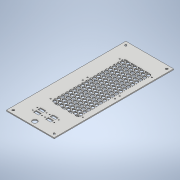
# Autodesk Inventor part: top_panel2
Saved by Autodesk Inventor 2022 (Build 260153000, 153)
## iProperties
Created: 2021-05-16
Part Number: top_panel2
Material: Generic
Document SubType Name: Modeling
Designer: gisen
Density: 1 g/cm^3
Appearance: Default
Author: gisen
Autodesk Inventor part; units mm, degrees
(part 1 of 2)
ref_plane "YZ Plane" through (0, 0, 0) normal (1, 0, 0) x (0, 1, 0)
ref_plane "XZ Plane" through (0, 0, 0) normal (0, 1, 0) x (-1, 0, 0)
ref_plane "XY Plane" through (0, 0, 0) normal (0, 0, 1) x (1, 0, 0)
sketch "Sketch1" plane through (0, 0, 0) normal (0, 0, 1) x (1, 0, 0)
  line L0 (-78, 195) -> (78, 195)
  line L1 (78, 195) -> (78, -195)
  line L2 (78, -195) -> (-78, -195)
  line L3 (-78, -195) -> (-78, 195)
  line L4 (-78, 195) -> (78, -195) construction
  line L5 (78, 195) -> (-78, -195) construction
  point P0 (0, 0)
  dimension "d1" = 156
  dimension "d2" = 390
  constraints: 12 end point, 2 midpoint, 2 parallel, 1 horizontal, 1 perpendicular
  measures "d1" distance of L0.start L0.end
  measures "d2" distance of L0.end L1.end
extrude "Extrusion1" add sketch "Sketch1" along normal blind 3
sketch "Sketch2" plane through (0, 0, 3) normal (0, 0, 1) x (1, 0, 0)
  line L0 (-78, -195) -> (78, -195) projected
  line L1 (-78, 195) -> (-78, -195) projected
  arc A0 (-64.4298, -185.2577) -> (-68.2577, -181.4298) centre (-66, -183) ccw
  arc A1 (-69.8472, -183.7153) -> (-66.7153, -186.8472) centre (-68, -185) ccw
  line L2 (-66.7153, -186.8472) -> (-64.4298, -185.2577)
  line L3 (-69.8472, -183.7153) -> (-68.2577, -181.4298)
  line L4 (0, 16.0888) -> (0, -25.3045)
  line L5 (-19.6832, 0) -> (22.709, 0)
  arc A2 (68.2577, -181.4298) -> (64.4298, -185.2577) centre (66, -183) ccw
  arc A3 (66.7153, -186.8472) -> (69.8472, -183.7153) centre (68, -185) ccw
  line L6 (66.7153, -186.8472) -> (64.4298, -185.2577)
  line L7 (69.8472, -183.7153) -> (68.2577, -181.4298)
  arc A4 (-68.2577, 181.4298) -> (-64.4298, 185.2577) centre (-66, 183) ccw
  arc A5 (-66.7153, 186.8472) -> (-69.8472, 183.7153) centre (-68, 185) ccw
  line L8 (-66.7153, 186.8472) -> (-64.4298, 185.2577)
  line L9 (-69.8472, 183.7153) -> (-68.2577, 181.4298)
  arc A6 (64.4298, 185.2577) -> (68.2577, 181.4298) centre (66, 183) ccw
  arc A7 (69.8472, 183.7153) -> (66.7153, 186.8472) centre (68, 185) ccw
  line L10 (66.7153, 186.8472) -> (64.4298, 185.2577)
  line L11 (69.8472, 183.7153) -> (68.2577, 181.4298)
  point P0 (0, 0)
  dimension "d11" = 12
  dimension "d12" = 10
  dimension "d13" = 12
  dimension "d14" = 10
  dimension "d15" = 5.5
  dimension "d16" = 4.5
  constraints: 24 symmetric about line, 20 end point, 16 point on circle, 8 centre point, 8 coincident, 4 tangent, 1 horizontal, 1 vertical, 6 other
  measures "d11" distance from line of L0 point (-66, -183)
  measures "d12" distance from line of L0 point (-68, -185)
  measures "d13" distance from line of L1 point (-66, -183)
  measures "d14" distance from line of L1 point (-68, -185)
  measures "d15" diameter of A0
  measures "d16" diameter of A1
extrude "Extrusion2" cut sketch "Sketch2" against normal up to surface (3 mm away)
sketch "Sketch4" plane through (0, 0, 3) normal (0, 0, 1) x (1, 0, 0)
  line L0 (-28.5, -132.4667) -> (-11.5, -132.4667)
  line L1 (-11.5, -132.4667) -> (-11.5, -141.4667)
  line L2 (-11.5, -141.4667) -> (-28.5, -141.4667)
  line L3 (-28.5, -141.4667) -> (-28.5, -132.4667)
  line L4 (-28.5, -132.4667) -> (-11.5, -141.4667) construction
  line L5 (-11.5, -132.4667) -> (-28.5, -141.4667) construction
  circle A0 centre (-35, -136.9667) radius 1.65
  circle A1 centre (-5, -136.9667) radius 1.65
  line L6 (0, -132.1595) -> (0, -155.449)
  line L7 (28.5, -132.4667) -> (11.5, -132.4667)
  line L8 (11.5, -132.4667) -> (11.5, -141.4667)
  line L9 (11.5, -141.4667) -> (28.5, -141.4667)
  line L10 (28.5, -141.4667) -> (28.5, -132.4667)
  line L11 (28.5, -132.4667) -> (11.5, -141.4667) construction
  line L12 (11.5, -132.4667) -> (28.5, -141.4667) construction
  circle A2 centre (35, -136.9667) radius 1.65
  circle A3 centre (5, -136.9667) radius 1.65
  line L13 (-30.7879, -144.4667) -> (-3.35, -144.4667)
  line L14 (-28.5, -156.4667) -> (-11.5, -156.4667)
  line L15 (-11.5, -156.4667) -> (-11.5, -147.4667)
  line L16 (-11.5, -147.4667) -> (-28.5, -147.4667)
  line L17 (-28.5, -147.4667) -> (-28.5, -156.4667)
  line L18 (-28.5, -156.4667) -> (-11.5, -147.4667) construction
  line L19 (-11.5, -156.4667) -> (-28.5, -147.4667) construction
  circle A4 centre (-35, -151.9667) radius 1.65
  circle A5 centre (-5, -151.9667) radius 1.65
  line L20 (28.5, -156.4667) -> (11.5, -156.4667)
  line L21 (11.5, -156.4667) -> (11.5, -147.4667)
  line L22 (11.5, -147.4667) -> (28.5, -147.4667)
  line L23 (28.5, -147.4667) -> (28.5, -156.4667)
  line L24 (28.5, -156.4667) -> (11.5, -147.4667) construction
  line L25 (11.5, -156.4667) -> (28.5, -147.4667) construction
  circle A6 centre (35, -151.9667) radius 1.65
  circle A7 centre (5, -151.9667) radius 1.65
  line L26 (-66.7153, 186.8472) -> (-64.4298, 185.2577) projected
  arc A8 (-68.2577, 181.4298) -> (-64.4298, 185.2577) centre (-66, 183) ccw projected
  line L27 (-68.2577, 181.4298) -> (-69.8472, 183.7153) projected
  arc A9 (-66.7153, 186.8472) -> (-69.8472, 183.7153) centre (-68, 185) ccw projected
  arc A10 (69.8472, 183.7153) -> (66.7153, 186.8472) centre (68, 185) ccw projected
  line L28 (69.8472, 183.7153) -> (68.2577, 181.4298) projected
  arc A11 (64.4298, 185.2577) -> (68.2577, 181.4298) centre (66, 183) ccw projected
  line L29 (64.4298, 185.2577) -> (66.7153, 186.8472) projected
  line L30 (66.7153, -186.8472) -> (64.4298, -185.2577) projected
  arc A12 (68.2577, -181.4298) -> (64.4298, -185.2577) centre (66, -183) ccw projected
  line L31 (68.2577, -181.4298) -> (69.8472, -183.7153) projected
  arc A13 (66.7153, -186.8472) -> (69.8472, -183.7153) centre (68, -185) ccw projected
  arc A14 (-69.8472, -183.7153) -> (-66.7153, -186.8472) centre (-68, -185) ccw projected
  line L32 (-69.8472, -183.7153) -> (-68.2577, -181.4298) projected
  arc A15 (-64.4298, -185.2577) -> (-68.2577, -181.4298) centre (-66, -183) ccw projected
  line L33 (-64.4298, -185.2577) -> (-66.7153, -186.8472) projected
  line L34 (78, 195) -> (-78, 195) projected
  line L35 (-78, 195) -> (-78, -195) projected
  line L36 (-78, -195) -> (78, -195) projected
  line L37 (78, -195) -> (78, 195) projected
  line L38 (78, -195) -> (-78, -195) projected
  point P0 (0, 0)
  point P1 (-20, -136.9667)
  point P2 (-5, -136.9667)
  point P3 (20, -136.9667)
  point P4 (-20, -151.9667)
  point P5 (20, -151.9667)
  point P6 (0, -195)
  dimension "d37" = 17
  dimension "d38" = 9
  dimension "d39" = 6.5
  dimension "d40" = 4.5
  dimension "d41" = 3.3
  dimension "d42" = 6.5
  dimension "d43" = 4.5
  dimension "d44" = 3.3
  dimension "d45" = 5
  dimension "d46" = 3
  dimension "d55" = 0
  constraints: 52 end point, 27 symmetric about line, 9 midpoint, 8 centre point, 8 coincident, 2 horizontal, 2 parallel, 1 perpendicular, 1 vertical, 6 other
  measures "d37" distance of L1.end L2.end
  measures "d38" distance of L0.end L1.end
  measures "d39" distance from line of L3 point (-35, -136.967)
  measures "d40" distance from line of point (-35, -136.967) L0
  measures "d41" diameter of A0
  measures "d42" distance from line of point (-5, -136.967) L1
  measures "d43" distance from line of L0 point (-5, -136.967)
  measures "d44" diameter of A1
  measures "d45" horizontal distance of A1.centre point (0, 0)
  measures "d46" distance between parallel lines of L13 L2
  measures "d55" distance from line of point (0, -195) L6
extrude "Extrusion4" cut sketch "Sketch4" against normal up to surface (3 mm away) contours L0 L1 L2 L3 | A0 | A1 | L10 L9 L8 L7 | A2 | A3 | L17 L16 L15 L14 | A4 | A5 | L20 L21 L22 L23 | A6 | A7
sketch "Sketch5" plane through (0, 0, 3) normal (0, 0, 1) x (1, 0, 0)
  line L0 (-78, -195) -> (78, -195) projected
  line L1 (-2.4755, -172.54) -> (2.4755, -172.54)
  line L2 (-2.4755, -187.46) -> (2.4755, -187.46)
  arc A0 (-2.4755, -172.54) -> (-2.4755, -187.46) centre (0, -180) ccw
  arc A1 (2.4755, -187.46) -> (2.4755, -172.54) centre (0, -180) ccw
  point P0 (0, 0)
  dimension "d49" = 15
  dimension "d51" = 7.46
  dimension "d52" = 7.46
  constraints: 4 end point, 4 point on circle, 2 centre point, 2 horizontal, 1 coincident
  measures "d49" distance from line of L0 point (0, -180)
  measures "d51" distance from line of A0.centre L1
  measures "d52" distance from line of point (0, -180) L2
extrude "Extrusion5" cut sketch "Sketch5" against normal up to surface (3 mm away)
sketch "Sketch7" plane through (0, 0, 3) normal (0, 0, 1) x (1, 0, 0)
  circle A0 centre (-38, -90.5) radius 2
  line L0 (-2.4755, -172.54) -> (2.4755, -172.54) projected
  arc A1 (2.4755, -187.46) -> (2.4755, -172.54) centre (0, -180) ccw projected
  line L1 (2.4755, -187.46) -> (-2.4755, -187.46) projected
  arc A2 (-2.4755, -172.54) -> (-2.4755, -187.46) centre (0, -180) ccw projected
  line L2 (-11.5, -156.4667) -> (-28.5, -156.4667) projected
  line L3 (-28.5, -156.4667) -> (-28.5, -147.4667) projected
  line L4 (-28.5, -147.4667) -> (-11.5, -147.4667) projected
  line L5 (-11.5, -147.4667) -> (-11.5, -156.4667) projected
  line L6 (11.5, -147.4667) -> (28.5, -147.4667) projected
  line L7 (28.5, -147.4667) -> (28.5, -156.4667) projected
  line L8 (28.5, -156.4667) -> (11.5, -156.4667) projected
  line L9 (11.5, -156.4667) -> (11.5, -147.4667) projected
  line L10 (11.5, -132.4667) -> (28.5, -132.4667) projected
  line L11 (28.5, -132.4667) -> (28.5, -141.4667) projected
  line L12 (28.5, -141.4667) -> (11.5, -141.4667) projected
  line L13 (11.5, -141.4667) -> (11.5, -132.4667) projected
  circle A3 centre (35, -151.9667) radius 1.65 projected
  circle A4 centre (-35, -151.9667) radius 1.65 projected
  circle A5 centre (5, -136.9667) radius 1.65 projected
  circle A6 centre (-5, -136.9667) radius 1.65 projected
  circle A7 centre (-35, -136.9667) radius 1.65 projected
  circle A8 centre (35, -136.9667) radius 1.65 projected
  circle A9 centre (-5, -151.9667) radius 1.65 projected
  circle A10 centre (5, -151.9667) radius 1.65 projected
  line L14 (-11.5, -132.4667) -> (-11.5, -141.4667) projected
  line L15 (-11.5, -141.4667) -> (-28.5, -141.4667) projected
  line L16 (-28.5, -141.4667) -> (-28.5, -132.4667) projected
  line L17 (-28.5, -132.4667) -> (-11.5, -132.4667) projected
  line L18 (-66.7153, 186.8472) -> (-64.4298, 185.2577) projected
  arc A11 (-68.2577, 181.4298) -> (-64.4298, 185.2577) centre (-66, 183) ccw projected
  line L19 (-68.2577, 181.4298) -> (-69.8472, 183.7153) projected
  arc A12 (-66.7153, 186.8472) -> (-69.8472, 183.7153) centre (-68, 185) ccw projected
  arc A13 (69.8472, 183.7153) -> (66.7153, 186.8472) centre (68, 185) ccw projected
  line L20 (69.8472, 183.7153) -> (68.2577, 181.4298) projected
  arc A14 (64.4298, 185.2577) -> (68.2577, 181.4298) centre (66, 183) ccw projected
  line L21 (64.4298, 185.2577) -> (66.7153, 186.8472) projected
  line L22 (66.7153, -186.8472) -> (64.4298, -185.2577) projected
  arc A15 (68.2577, -181.4298) -> (64.4298, -185.2577) centre (66, -183) ccw projected
  line L23 (68.2577, -181.4298) -> (69.8472, -183.7153) projected
  arc A16 (66.7153, -186.8472) -> (69.8472, -183.7153) centre (68, -185) ccw projected
  arc A17 (-69.8472, -183.7153) -> (-66.7153, -186.8472) centre (-68, -185) ccw projected
  line L24 (-69.8472, -183.7153) -> (-68.2577, -181.4298) projected
  arc A18 (-64.4298, -185.2577) -> (-68.2577, -181.4298) centre (-66, -183) ccw projected
  line L25 (-64.4298, -185.2577) -> (-66.7153, -186.8472) projected
  line L26 (78, 195) -> (-78, 195) projected
  line L27 (-78, 195) -> (-78, -195) projected
  line L28 (-78, -195) -> (78, -195) projected
  line L29 (78, -195) -> (78, 195) projected
  circle A19 centre (-38, 14.5) radius 2
  circle A20 centre (-38, 30) radius 2
  circle A21 centre (-38, 135) radius 2
  line L30 (14.5, 19.3358) -> (14.5, -21.6)
  circle A22 centre (67, -90.5) radius 2
  circle A23 centre (67, 14.5) radius 2
  circle A24 centre (67, 30) radius 2
  circle A25 centre (67, 135) radius 2
  point P0 (0, 0)
  dimension "d56" = 4
  dimension "d57" = 40
  dimension "d60" = 4
  dimension "d61" = 105
  dimension "d62" = 40
  dimension "d63" = 4
  dimension "d65" = 40
  dimension "d66" = 4
  dimension "d68" = 40
  dimension "d69" = 60
  dimension "d103" = 15.5
  dimension "d104" = 105
  dimension "d112" = 52.5
  constraints: 8 centre point, 4 symmetric about line, 2 end point, 1 vertical, 4 other
  measures "d56" diameter of A0
  measures "d57" distance from line of L27 A0.centre
  measures "d60" diameter of A19
  measures "d61" distance of A0.centre A19.centre
  measures "d62" distance from line of L27 A19.centre
  measures "d63" diameter of A20
  measures "d65" distance from line of L27 A20.centre
  measures "d66" diameter of A21
  measures "d68" distance from line of L27 A21.centre
  measures "d69" distance from line of L26 A21.centre
  measures "d103" distance of A19.centre A20.centre
  measures "d104" distance of A21.centre A20.centre
  measures "d112" distance from line of A19.centre L30
extrude "Extrusion7" cut sketch "Sketch7" against normal up to surface (3 mm away) contours A0 | A19 | A20 | A21 | A22 | A23 | A24 | A25
sketch "Sketch8" plane through (0, 0, 3) normal (0, 0, 1) x (1, 0, 0)
  circle A0 centre (-38, -90.5) radius 2 projected
  circle A1 centre (-38, 14.5) radius 2 projected
  circle A2 centre (67, 30) radius 2 projected
  circle A3 centre (67, 135) radius 2 projected
  circle A4 centre (67, -90.5) radius 2 projected
  circle A5 centre (67, 14.5) radius 2 projected
  circle A6 centre (-38, 30) radius 2 projected
  circle A7 centre (-38, 135) radius 2 projected
  line L0 (-2.4755, -172.54) -> (2.4755, -172.54) projected
  arc A8 (2.4755, -187.46) -> (2.4755, -172.54) centre (0, -180) ccw projected
  line L1 (2.4755, -187.46) -> (-2.4755, -187.46) projected
  arc A9 (-2.4755, -172.54) -> (-2.4755, -187.46) centre (0, -180) ccw projected
  line L2 (-11.5, -156.4667) -> (-28.5, -156.4667) projected
  line L3 (-28.5, -156.4667) -> (-28.5, -147.4667) projected
  line L4 (-28.5, -147.4667) -> (-11.5, -147.4667) projected
  line L5 (-11.5, -147.4667) -> (-11.5, -156.4667) projected
  line L6 (11.5, -147.4667) -> (28.5, -147.4667) projected
  line L7 (28.5, -147.4667) -> (28.5, -156.4667) projected
  line L8 (28.5, -156.4667) -> (11.5, -156.4667) projected
  line L9 (11.5, -156.4667) -> (11.5, -147.4667) projected
  line L10 (11.5, -132.4667) -> (28.5, -132.4667) projected
  line L11 (28.5, -132.4667) -> (28.5, -141.4667) projected
  line L12 (28.5, -141.4667) -> (11.5, -141.4667) projected
  line L13 (11.5, -141.4667) -> (11.5, -132.4667) projected
  circle A10 centre (35, -151.9667) radius 1.65 projected
  circle A11 centre (-35, -151.9667) radius 1.65 projected
  circle A12 centre (5, -136.9667) radius 1.65 projected
  circle A13 centre (-5, -136.9667) radius 1.65 projected
  circle A14 centre (-35, -136.9667) radius 1.65 projected
  circle A15 centre (35, -136.9667) radius 1.65 projected
  circle A16 centre (-5, -151.9667) radius 1.65 projected
  circle A17 centre (5, -151.9667) radius 1.65 projected
  line L14 (-11.5, -132.4667) -> (-11.5, -141.4667) projected
  line L15 (-11.5, -141.4667) -> (-28.5, -141.4667) projected
  line L16 (-28.5, -141.4667) -> (-28.5, -132.4667) projected
  line L17 (-28.5, -132.4667) -> (-11.5, -132.4667) projected
  line L18 (-66.7153, 186.8472) -> (-64.4298, 185.2577) projected
  arc A18 (-68.2577, 181.4298) -> (-64.4298, 185.2577) centre (-66, 183) ccw projected
  line L19 (-68.2577, 181.4298) -> (-69.8472, 183.7153) projected
  arc A19 (-66.7153, 186.8472) -> (-69.8472, 183.7153) centre (-68, 185) ccw projected
  arc A20 (69.8472, 183.7153) -> (66.7153, 186.8472) centre (68, 185) ccw projected
  line L20 (69.8472, 183.7153) -> (68.2577, 181.4298) projected
  arc A21 (64.4298, 185.2577) -> (68.2577, 181.4298) centre (66, 183) ccw projected
  line L21 (64.4298, 185.2577) -> (66.7153, 186.8472) projected
  line L22 (66.7153, -186.8472) -> (64.4298, -185.2577) projected
  arc A22 (68.2577, -181.4298) -> (64.4298, -185.2577) centre (66, -183) ccw projected
  line L23 (68.2577, -181.4298) -> (69.8472, -183.7153) projected
  arc A23 (66.7153, -186.8472) -> (69.8472, -183.7153) centre (68, -185) ccw projected
  arc A24 (-69.8472, -183.7153) -> (-66.7153, -186.8472) centre (-68, -185) ccw projected
  line L24 (-69.8472, -183.7153) -> (-68.2577, -181.4298) projected
  arc A25 (-64.4298, -185.2577) -> (-68.2577, -181.4298) centre (-66, -183) ccw projected
  line L25 (-64.4298, -185.2577) -> (-66.7153, -186.8472) projected
  line L26 (78, 195) -> (-78, 195) projected
  line L27 (-78, 195) -> (-78, -195) projected
  line L28 (-78, -195) -> (78, -195) projected
  line L29 (78, -195) -> (78, 195) projected
  circle A26 centre (-38, 135) radius 2 projected
  circle A27 centre (-38, 135) radius 6.33
  line L30 (-31.67, 135) -> (-31.67, 13.6115)
  arc A28 (-24.17, 142.5) -> (-31.67, 135) centre (-24.17, 135) ccw
  line L31 (-31.67, 13.6115) -> (-31.67, -90.5)
  arc A29 (-31.67, -90.5) -> (-24.17, -98) centre (-24.17, -90.5) ccw
  line L32 (-24.17, -98) -> (-10.2337, -98)
  line L33 (-24.17, 142.5) -> (-11.5, 142.5)
  line L34 (14.5, 11.7665) -> (14.5, -13.3152)
  line L35 (60.67, 135) -> (60.67, 13.6115)
  arc A30 (60.67, 135) -> (53.17, 142.5) centre (53.17, 135) ccw
  line L36 (60.67, 13.6115) -> (60.67, -90.5)
  arc A31 (53.17, -98) -> (60.67, -90.5) centre (53.17, -90.5) ccw
  line L37 (53.17, -98) -> (39.2337, -98)
  line L38 (53.17, 142.5) -> (40.5, 142.5)
  line L39 (40.5, 142.5) -> (-11.5, 142.5)
  line L40 (39.2337, -98) -> (12.6121, -98)
  circle A32 centre (-38, -90.5) radius 2 projected
  line L41 (-10.2337, -98) -> (21.6365, -98)
  line L42 (-21.286, -85.5048) -> (-27.054, -85.5048)
  line L43 (-27.054, -85.5048) -> (-29.9379, -90.5)
  line L44 (-29.9379, -90.5) -> (-27.054, -95.4952)
  line L45 (-27.054, -95.4952) -> (-21.286, -95.4952)
  line L46 (-21.286, -95.4952) -> (-18.4021, -90.5)
  line L47 (-18.4021, -90.5) -> (-21.286, -85.5048)
  line L48 (-7.1521, -84.0048) -> (-10.036, -89)
  line L49 (-10.036, -89) -> (-15.804, -89)
  line L50 (-15.804, -89) -> (-18.6879, -84.0048)
  line L51 (-7.1521, -96.9952) -> (-10.036, -92)
  line L52 (-10.036, -92) -> (-15.804, -92)
  line L53 (-15.804, -92) -> (-18.6879, -96.9952)
  line L54 (-1.67, -85.5048) -> (-4.554, -85.5048)
  line L55 (-4.554, -85.5048) -> (-7.4379, -90.5)
  line L56 (-7.4379, -90.5) -> (-4.554, -95.4952)
  line L57 (-4.554, -95.4952) -> (-1.67, -95.4952)
  line L58 (17.946, -85.5048) -> (20.83, -85.5048)
  line L59 (20.83, -95.4952) -> (17.946, -95.4952)
  line L60 (17.946, -95.4952) -> (15.0621, -90.5)
  line L61 (15.0621, -90.5) -> (17.946, -85.5048)
  line L62 (3.8121, -84.0048) -> (6.696, -89)
  line L63 (6.696, -89) -> (12.464, -89)
  line L64 (12.464, -89) -> (15.3479, -84.0048)
  line L65 (3.8121, -96.9952) -> (6.696, -92)
  line L66 (6.696, -92) -> (12.464, -92)
  line L67 (12.464, -92) -> (15.3479, -96.9952)
  line L68 (-1.67, -85.5048) -> (1.214, -85.5048)
  line L69 (1.214, -85.5048) -> (4.0979, -90.5)
  line L70 (4.0979, -90.5) -> (1.214, -95.4952)
  line L71 (1.214, -95.4952) -> (-1.67, -95.4952)
  line L72 (62.946, -95.4952) -> (60.0621, -90.5)
  line L73 (60.0621, -90.5) -> (62.946, -85.5048)
  line L74 (48.8121, -84.0048) -> (51.696, -89)
  line L75 (51.696, -89) -> (57.464, -89)
  line L76 (57.464, -89) -> (60.3479, -84.0048)
  line L77 (48.8121, -96.9952) -> (51.696, -92)
  line L78 (51.696, -92) -> (57.464, -92)
  line L79 (57.464, -92) -> (60.3479, -96.9952)
  line L80 (43.33, -85.5048) -> (46.214, -85.5048)
  line L81 (46.214, -85.5048) -> (49.0979, -90.5)
  line L82 (49.0979, -90.5) -> (46.214, -95.4952)
  line L83 (46.214, -95.4952) -> (43.33, -95.4952)
  line L84 (37.8479, -96.9952) -> (34.964, -92)
  line L85 (37.5621, -90.5) -> (40.446, -95.4952)
  line L86 (43.33, -85.5048) -> (40.446, -85.5048)
  line L87 (40.446, -85.5048) -> (37.5621, -90.5)
  line L88 (37.8479, -84.0048) -> (34.964, -89)
  line L89 (34.964, -92) -> (29.196, -92)
  line L90 (34.964, -89) -> (29.196, -89)
  line L91 (29.196, -92) -> (26.3121, -96.9952)
  line L92 (40.446, -95.4952) -> (43.33, -95.4952)
  line L93 (23.714, -95.4952) -> (26.5979, -90.5)
  line L94 (29.196, -89) -> (26.3121, -84.0048)
  line L95 (26.5979, -90.5) -> (23.714, -85.5048)
  line L96 (23.714, -85.5048) -> (20.83, -85.5048)
  line L97 (20.83, -95.4952) -> (23.714, -95.4952)
  line L98 (-21.286, -82.5048) -> (-27.054, -82.5048)
  line L99 (-27.054, -82.5048) -> (-29.9379, -77.5096)
  line L100 (-29.9379, -77.5096) -> (-27.054, -72.5144)
  line L101 (-27.054, -72.5144) -> (-21.286, -72.5144)
  line L102 (-21.286, -72.5144) -> (-18.4021, -77.5096)
  line L103 (-18.4021, -77.5096) -> (-21.286, -82.5048)
  line L104 (-7.1521, -84.0048) -> (-10.036, -79.0096)
  line L105 (-10.036, -79.0096) -> (-15.804, -79.0096)
  line L106 (-15.804, -79.0096) -> (-18.6879, -84.0048)
  line L107 (-7.1521, -71.0144) -> (-10.036, -76.0096)
  line L108 (-10.036, -76.0096) -> (-15.804, -76.0096)
  line L109 (-15.804, -76.0096) -> (-18.6879, -71.0144)
  line L110 (-1.67, -82.5048) -> (-4.554, -82.5048)
  line L111 (-4.554, -82.5048) -> (-7.4379, -77.5096)
  line L112 (-7.4379, -77.5096) -> (-4.554, -72.5144)
  line L113 (-4.554, -72.5144) -> (-1.67, -72.5144)
  line L114 (3.8121, -71.0144) -> (6.696, -76.0096)
  line L115 (4.0979, -77.5096) -> (1.214, -72.5144)
  line L116 (-1.67, -82.5048) -> (1.214, -82.5048)
  line L117 (1.214, -82.5048) -> (4.0979, -77.5096)
  line L118 (3.8121, -84.0048) -> (6.696, -79.0096)
  line L119 (6.696, -76.0096) -> (12.464, -76.0096)
  line L120 (6.696, -79.0096) -> (12.464, -79.0096)
  line L121 (12.464, -76.0096) -> (15.3479, -71.0144)
  line L122 (1.214, -72.5144) -> (-1.67, -72.5144)
  line L123 (17.946, -72.5144) -> (15.0621, -77.5096)
  line L124 (12.464, -79.0096) -> (15.3479, -84.0048)
  line L125 (15.0621, -77.5096) -> (17.946, -82.5048)
  line L126 (17.946, -82.5048) -> (20.83, -82.5048)
  line L127 (20.83, -72.5144) -> (17.946, -72.5144)
  line L128 (23.714, -82.5048) -> (20.83, -82.5048)
  line L129 (60.0621, -77.5096) -> (62.946, -82.5048)
  line L130 (57.464, -79.0096) -> (60.3479, -84.0048)
  line L131 (62.946, -72.5144) -> (60.0621, -77.5096)
  line L132 (57.464, -76.0096) -> (60.3479, -71.0144)
  line L133 (51.696, -76.0096) -> (57.464, -76.0096)
  line L134 (51.696, -79.0096) -> (57.464, -79.0096)
  line L135 (37.8479, -71.0144) -> (34.964, -76.0096)
  line L136 (34.964, -76.0096) -> (29.196, -76.0096)
  line L137 (34.964, -79.0096) -> (29.196, -79.0096)
  line L138 (37.8479, -84.0048) -> (34.964, -79.0096)
  line L139 (40.446, -82.5048) -> (37.5621, -77.5096)
  line L140 (37.5621, -77.5096) -> (40.446, -72.5144)
  line L141 (43.33, -82.5048) -> (40.446, -82.5048)
  line L142 (20.83, -72.5144) -> (23.714, -72.5144)
  line L143 (29.196, -76.0096) -> (26.3121, -71.0144)
  line L144 (23.714, -72.5144) -> (26.5979, -77.5096)
  line L145 (29.196, -79.0096) -> (26.3121, -84.0048)
  line L146 (26.5979, -77.5096) -> (23.714, -82.5048)
  line L147 (48.8121, -84.0048) -> (51.696, -79.0096)
  line L148 (48.8121, -71.0144) -> (51.696, -76.0096)
  line L149 (46.214, -82.5048) -> (49.0979, -77.5096)
  line L150 (49.0979, -77.5096) -> (46.214, -72.5144)
  line L151 (46.214, -72.5144) -> (43.33, -72.5144)
  line L152 (40.446, -72.5144) -> (43.33, -72.5144)
  line L153 (43.33, -82.5048) -> (46.214, -82.5048)
  line L154 (-32.969, -89.75) -> (-29.6521, -84.0048)
  line L155 (-29.6521, -84.0048) -> (-33.4021, -77.5096)
  line L156 (-33.4021, -77.5096) -> (-29.6521, -71.0144)
  line L157 (-21.286, -56.524) -> (-27.054, -56.524)
  line L158 (-27.054, -56.524) -> (-29.9379, -51.5289)
  line L159 (-29.9379, -51.5289) -> (-27.054, -46.5337)
  line L160 (-27.054, -46.5337) -> (-21.286, -46.5337)
  line L161 (-21.286, -46.5337) -> (-18.4021, -51.5289)
  line L162 (-18.4021, -51.5289) -> (-21.286, -56.524)
  line L163 (-7.1521, -58.024) -> (-10.036, -53.0289)
  line L164 (-10.036, -53.0289) -> (-15.804, -53.0289)
  line L165 (-15.804, -53.0289) -> (-18.6879, -58.024)
  line L166 (-7.1521, -45.0337) -> (-10.036, -50.0289)
  line L167 (-10.036, -50.0289) -> (-15.804, -50.0289)
  line L168 (-15.804, -50.0289) -> (-18.6879, -45.0337)
  line L169 (-1.67, -56.524) -> (-4.554, -56.524)
  line L170 (-4.554, -56.524) -> (-7.4379, -51.5289)
  line L171 (-7.4379, -51.5289) -> (-4.554, -46.5337)
  line L172 (-4.554, -46.5337) -> (-1.67, -46.5337)
  line L173 (3.8121, -45.0337) -> (6.696, -50.0289)
  line L174 (4.0979, -51.5289) -> (1.214, -46.5337)
  line L175 (-1.67, -56.524) -> (1.214, -56.524)
  line L176 (1.214, -56.524) -> (4.0979, -51.5289)
  line L177 (3.8121, -58.024) -> (6.696, -53.0289)
  line L178 (6.696, -50.0289) -> (12.464, -50.0289)
  line L179 (6.696, -53.0289) -> (12.464, -53.0289)
  line L180 (12.464, -50.0289) -> (15.3479, -45.0337)
  line L181 (1.214, -46.5337) -> (-1.67, -46.5337)
  line L182 (17.946, -46.5337) -> (15.0621, -51.5289)
  line L183 (12.464, -53.0289) -> (15.3479, -58.024)
  line L184 (15.0621, -51.5289) -> (17.946, -56.524)
  line L185 (17.946, -56.524) -> (20.83, -56.524)
  line L186 (20.83, -46.5337) -> (17.946, -46.5337)
  line L187 (23.714, -56.524) -> (20.83, -56.524)
  line L188 (60.0621, -51.5289) -> (62.946, -56.524)
  line L189 (57.464, -53.0289) -> (60.3479, -58.024)
  line L190 (62.946, -46.5337) -> (60.0621, -51.5289)
  line L191 (57.464, -50.0289) -> (60.3479, -45.0337)
  line L192 (51.696, -50.0289) -> (57.464, -50.0289)
  line L193 (51.696, -53.0289) -> (57.464, -53.0289)
  line L194 (37.8479, -45.0337) -> (34.964, -50.0289)
  line L195 (34.964, -50.0289) -> (29.196, -50.0289)
  line L196 (34.964, -53.0289) -> (29.196, -53.0289)
  line L197 (37.8479, -58.024) -> (34.964, -53.0289)
  line L198 (40.446, -56.524) -> (37.5621, -51.5289)
  line L199 (37.5621, -51.5289) -> (40.446, -46.5337)
  line L200 (43.33, -56.524) -> (40.446, -56.524)
  line L201 (20.83, -46.5337) -> (23.714, -46.5337)
  line L202 (29.196, -50.0289) -> (26.3121, -45.0337)
  line L203 (23.714, -46.5337) -> (26.5979, -51.5289)
  line L204 (29.196, -53.0289) -> (26.3121, -58.024)
  line L205 (26.5979, -51.5289) -> (23.714, -56.524)
  line L206 (48.8121, -58.024) -> (51.696, -53.0289)
  line L207 (48.8121, -45.0337) -> (51.696, -50.0289)
  line L208 (46.214, -56.524) -> (49.0979, -51.5289)
  line L209 (49.0979, -51.5289) -> (46.214, -46.5337)
  line L210 (46.214, -46.5337) -> (43.33, -46.5337)
  line L211 (40.446, -46.5337) -> (43.33, -46.5337)
  line L212 (43.33, -56.524) -> (46.214, -56.524)
  line L213 (-18.4021, -64.5192) -> (-21.286, -59.524)
  line L214 (-21.286, -69.5144) -> (-18.4021, -64.5192)
  line L215 (-27.054, -69.5144) -> (-21.286, -69.5144)
  line L216 (-21.286, -59.524) -> (-27.054, -59.524)
  line L217 (-15.804, -66.0192) -> (-18.6879, -71.0144)
  line L218 (-10.036, -66.0192) -> (-15.804, -66.0192)
  line L219 (-10.036, -63.0192) -> (-15.804, -63.0192)
  line L220 (-7.1521, -71.0144) -> (-10.036, -66.0192)
  line L221 (-7.4379, -64.5192) -> (-4.554, -69.5144)
  line L222 (-7.1521, -58.024) -> (-10.036, -63.0192)
  line L223 (-4.554, -59.524) -> (-7.4379, -64.5192)
  line L224 (-15.804, -63.0192) -> (-18.6879, -58.024)
  line L225 (-1.67, -59.524) -> (-4.554, -59.524)
  line L226 (-4.554, -69.5144) -> (-1.67, -69.5144)
  line L227 (1.214, -69.5144) -> (-1.67, -69.5144)
  line L228 (-1.67, -59.524) -> (1.214, -59.524)
  line L229 (4.0979, -64.5192) -> (1.214, -69.5144)
  line L230 (3.8121, -71.0144) -> (6.696, -66.0192)
  line L231 (1.214, -59.524) -> (4.0979, -64.5192)
  line L232 (3.8121, -58.024) -> (6.696, -63.0192)
  line L233 (17.946, -59.524) -> (20.83, -59.524)
  line L234 (12.464, -63.0192) -> (15.3479, -58.024)
  line L235 (6.696, -63.0192) -> (12.464, -63.0192)
  line L236 (15.0621, -64.5192) -> (17.946, -59.524)
  line L237 (6.696, -66.0192) -> (12.464, -66.0192)
  line L238 (17.946, -69.5144) -> (15.0621, -64.5192)
  line L239 (12.464, -66.0192) -> (15.3479, -71.0144)
  line L240 (20.83, -69.5144) -> (17.946, -69.5144)
  line L241 (51.696, -63.0192) -> (57.464, -63.0192)
  line L242 (51.696, -66.0192) -> (57.464, -66.0192)
  line L243 (20.83, -69.5144) -> (23.714, -69.5144)
  line L244 (23.714, -59.524) -> (20.83, -59.524)
  line L245 (23.714, -69.5144) -> (26.5979, -64.5192)
  line L246 (26.5979, -64.5192) -> (23.714, -59.524)
  line L247 (29.196, -63.0192) -> (26.3121, -58.024)
  line L248 (29.196, -66.0192) -> (26.3121, -71.0144)
  line L249 (34.964, -63.0192) -> (29.196, -63.0192)
  line L250 (34.964, -66.0192) -> (29.196, -66.0192)
  line L251 (37.8479, -58.024) -> (34.964, -63.0192)
  line L252 (37.8479, -71.0144) -> (34.964, -66.0192)
  line L253 (48.8121, -71.0144) -> (51.696, -66.0192)
  line L254 (48.8121, -58.024) -> (51.696, -63.0192)
  line L255 (46.214, -59.524) -> (49.0979, -64.5192)
  line L256 (49.0979, -64.5192) -> (46.214, -69.5144)
  line L257 (43.33, -59.524) -> (46.214, -59.524)
  line L258 (46.214, -69.5144) -> (43.33, -69.5144)
  line L259 (43.33, -59.524) -> (40.446, -59.524)
  line L260 (40.446, -59.524) -> (37.5621, -64.5192)
  line L261 (40.446, -69.5144) -> (43.33, -69.5144)
  line L262 (37.5621, -64.5192) -> (40.446, -69.5144)
  line L263 (57.464, -66.0192) -> (60.3479, -71.0144)
  line L264 (57.464, -63.0192) -> (60.3479, -58.024)
  line L265 (60.0621, -64.5192) -> (62.946, -59.524)
  line L266 (62.946, -69.5144) -> (60.0621, -64.5192)
  line L267 (-27.054, -59.524) -> (-29.9379, -64.5192)
  line L268 (-29.9379, -64.5192) -> (-27.054, -69.5144)
  line L269 (-32.969, -52.2789) -> (-29.6521, -58.024)
  line L270 (-29.6521, -58.024) -> (-33.4021, -64.5192)
  line L271 (-33.4021, -64.5192) -> (-29.6521, -71.0144)
  line L272 (-21.286, -4.5625) -> (-27.054, -4.5625)
  line L273 (-27.054, -4.5625) -> (-29.9379, 0.4327)
  line L274 (-29.9379, 0.4327) -> (-27.054, 5.4279)
  line L275 (-27.054, 5.4279) -> (-21.286, 5.4279)
  line L276 (-21.286, 5.4279) -> (-18.4021, 0.4327)
  line L277 (-18.4021, 0.4327) -> (-21.286, -4.5625)
  line L278 (-7.1521, -6.0625) -> (-10.036, -1.0673)
  line L279 (-10.036, -1.0673) -> (-15.804, -1.0673)
  line L280 (-15.804, -1.0673) -> (-18.6879, -6.0625)
  line L281 (-7.1521, 6.9279) -> (-10.036, 1.9327)
  line L282 (-10.036, 1.9327) -> (-15.804, 1.9327)
  line L283 (-15.804, 1.9327) -> (-18.6879, 6.9279)
  line L284 (-1.67, -4.5625) -> (-4.554, -4.5625)
  line L285 (-4.554, -4.5625) -> (-7.4379, 0.4327)
  line L286 (-7.4379, 0.4327) -> (-4.554, 5.4279)
  line L287 (-4.554, 5.4279) -> (-1.67, 5.4279)
  line L288 (3.8121, 6.9279) -> (6.696, 1.9327)
  line L289 (4.0979, 0.4327) -> (1.214, 5.4279)
  line L290 (-1.67, -4.5625) -> (1.214, -4.5625)
  line L291 (1.214, -4.5625) -> (4.0979, 0.4327)
  line L292 (3.8121, -6.0625) -> (6.696, -1.0673)
  line L293 (6.696, 1.9327) -> (12.464, 1.9327)
  line L294 (6.696, -1.0673) -> (12.464, -1.0673)
  line L295 (12.464, 1.9327) -> (15.3479, 6.9279)
  line L296 (1.214, 5.4279) -> (-1.67, 5.4279)
  line L297 (17.946, 5.4279) -> (15.0621, 0.4327)
  line L298 (12.464, -1.0673) -> (15.3479, -6.0625)
  line L299 (15.0621, 0.4327) -> (17.946, -4.5625)
  line L300 (17.946, -4.5625) -> (20.83, -4.5625)
  line L301 (20.83, 5.4279) -> (17.946, 5.4279)
  line L302 (23.714, -4.5625) -> (20.83, -4.5625)
  line L303 (60.0621, 0.4327) -> (62.946, -4.5625)
  line L304 (57.464, -1.0673) -> (60.3479, -6.0625)
  line L305 (62.946, 5.4279) -> (60.0621, 0.4327)
  line L306 (57.464, 1.9327) -> (60.3479, 6.9279)
  line L307 (51.696, 1.9327) -> (57.464, 1.9327)
  line L308 (51.696, -1.0673) -> (57.464, -1.0673)
  line L309 (37.8479, 6.9279) -> (34.964, 1.9327)
  line L310 (34.964, 1.9327) -> (29.196, 1.9327)
  line L311 (34.964, -1.0673) -> (29.196, -1.0673)
  line L312 (37.8479, -6.0625) -> (34.964, -1.0673)
  line L313 (40.446, -4.5625) -> (37.5621, 0.4327)
  line L314 (37.5621, 0.4327) -> (40.446, 5.4279)
  line L315 (43.33, -4.5625) -> (40.446, -4.5625)
  line L316 (20.83, 5.4279) -> (23.714, 5.4279)
  line L317 (29.196, 1.9327) -> (26.3121, 6.9279)
  line L318 (23.714, 5.4279) -> (26.5979, 0.4327)
  line L319 (29.196, -1.0673) -> (26.3121, -6.0625)
  line L320 (26.5979, 0.4327) -> (23.714, -4.5625)
  line L321 (48.8121, -6.0625) -> (51.696, -1.0673)
  line L322 (48.8121, 6.9279) -> (51.696, 1.9327)
  line L323 (46.214, -4.5625) -> (49.0979, 0.4327)
  line L324 (49.0979, 0.4327) -> (46.214, 5.4279)
  line L325 (46.214, 5.4279) -> (43.33, 5.4279)
  line L326 (40.446, 5.4279) -> (43.33, 5.4279)
  line L327 (43.33, -4.5625) -> (46.214, -4.5625)
  line L328 (-18.4021, -12.5577) -> (-21.286, -7.5625)
  line L329 (-21.286, -17.5529) -> (-18.4021, -12.5577)
  line L330 (-27.054, -17.5529) -> (-21.286, -17.5529)
  line L331 (-21.286, -7.5625) -> (-27.054, -7.5625)
  line L332 (-15.804, -14.0577) -> (-18.6879, -19.0529)
  line L333 (-10.036, -14.0577) -> (-15.804, -14.0577)
  line L334 (-10.036, -11.0577) -> (-15.804, -11.0577)
  line L335 (-7.1521, -19.0529) -> (-10.036, -14.0577)
  line L336 (-7.4379, -12.5577) -> (-4.554, -17.5529)
  line L337 (-7.1521, -6.0625) -> (-10.036, -11.0577)
  line L338 (-4.554, -7.5625) -> (-7.4379, -12.5577)
  line L339 (-15.804, -11.0577) -> (-18.6879, -6.0625)
  line L340 (-1.67, -7.5625) -> (-4.554, -7.5625)
  line L341 (-4.554, -17.5529) -> (-1.67, -17.5529)
  line L342 (1.214, -17.5529) -> (-1.67, -17.5529)
  line L343 (-1.67, -7.5625) -> (1.214, -7.5625)
  line L344 (4.0979, -12.5577) -> (1.214, -17.5529)
  line L345 (3.8121, -19.0529) -> (6.696, -14.0577)
  line L346 (1.214, -7.5625) -> (4.0979, -12.5577)
  line L347 (3.8121, -6.0625) -> (6.696, -11.0577)
  line L348 (17.946, -7.5625) -> (20.83, -7.5625)
  line L349 (12.464, -11.0577) -> (15.3479, -6.0625)
  line L350 (6.696, -11.0577) -> (12.464, -11.0577)
  line L351 (15.0621, -12.5577) -> (17.946, -7.5625)
  line L352 (6.696, -14.0577) -> (12.464, -14.0577)
  line L353 (17.946, -17.5529) -> (15.0621, -12.5577)
  line L354 (12.464, -14.0577) -> (15.3479, -19.0529)
  line L355 (20.83, -17.5529) -> (17.946, -17.5529)
  line L356 (51.696, -11.0577) -> (57.464, -11.0577)
  line L357 (51.696, -14.0577) -> (57.464, -14.0577)
  line L358 (20.83, -17.5529) -> (23.714, -17.5529)
  line L359 (23.714, -7.5625) -> (20.83, -7.5625)
  line L360 (23.714, -17.5529) -> (26.5979, -12.5577)
  line L361 (26.5979, -12.5577) -> (23.714, -7.5625)
  line L362 (29.196, -11.0577) -> (26.3121, -6.0625)
  line L363 (29.196, -14.0577) -> (26.3121, -19.0529)
  line L364 (34.964, -11.0577) -> (29.196, -11.0577)
  line L365 (34.964, -14.0577) -> (29.196, -14.0577)
  line L366 (37.8479, -6.0625) -> (34.964, -11.0577)
  line L367 (37.8479, -19.0529) -> (34.964, -14.0577)
  line L368 (48.8121, -19.0529) -> (51.696, -14.0577)
  line L369 (48.8121, -6.0625) -> (51.696, -11.0577)
  line L370 (46.214, -7.5625) -> (49.0979, -12.5577)
  line L371 (49.0979, -12.5577) -> (46.214, -17.5529)
  line L372 (43.33, -7.5625) -> (46.214, -7.5625)
  line L373 (46.214, -17.5529) -> (43.33, -17.5529)
  line L374 (43.33, -7.5625) -> (40.446, -7.5625)
  line L375 (40.446, -7.5625) -> (37.5621, -12.5577)
  line L376 (40.446, -17.5529) -> (43.33, -17.5529)
  line L377 (37.5621, -12.5577) -> (40.446, -17.5529)
  line L378 (57.464, -14.0577) -> (60.3479, -19.0529)
  line L379 (57.464, -11.0577) -> (60.3479, -6.0625)
  line L380 (60.0621, -12.5577) -> (62.946, -7.5625)
  line L381 (62.946, -17.5529) -> (60.0621, -12.5577)
  line L382 (-27.054, -7.5625) -> (-29.9379, -12.5577)
  line L383 (-29.9379, -12.5577) -> (-27.054, -17.5529)
  line L384 (-32.969, -0.3173) -> (-29.6521, -6.0625)
  line L385 (-29.6521, -6.0625) -> (-33.4021, -12.5577)
  line L386 (-33.4021, -12.5577) -> (-29.6521, -19.0529)
  line L387 (-15.804, -27.0481) -> (-18.6879, -32.0433)
  line L388 (-18.4021, -25.5481) -> (-21.286, -30.5433)
  line L389 (-21.286, -30.5433) -> (-27.054, -30.5433)
  line L390 (-18.4021, -38.5385) -> (-21.286, -33.5433)
  line L391 (-27.054, -30.5433) -> (-29.9379, -25.5481)
  line L392 (-29.6521, -32.0433) -> (-33.4021, -25.5481)
  line L393 (-32.969, -37.7885) -> (-29.6521, -32.0433)
  line L394 (-27.054, -33.5433) -> (-29.9379, -38.5385)
  line L395 (-21.286, -33.5433) -> (-27.054, -33.5433)
  line L396 (23.714, -43.5337) -> (26.5979, -38.5385)
  line L397 (26.5979, -38.5385) -> (23.714, -33.5433)
  line L398 (29.196, -40.0385) -> (26.3121, -45.0337)
  line L399 (29.196, -37.0385) -> (26.3121, -32.0433)
  line L400 (34.964, -37.0385) -> (29.196, -37.0385)
  line L401 (34.964, -40.0385) -> (29.196, -40.0385)
  line L402 (37.8479, -32.0433) -> (34.964, -37.0385)
  line L403 (37.8479, -45.0337) -> (34.964, -40.0385)
  line L404 (23.714, -33.5433) -> (20.83, -33.5433)
  line L405 (20.83, -43.5337) -> (23.714, -43.5337)
  line L406 (20.83, -43.5337) -> (17.946, -43.5337)
  line L407 (17.946, -33.5433) -> (20.83, -33.5433)
  line L408 (17.946, -43.5337) -> (15.0621, -38.5385)
  line L409 (15.0621, -38.5385) -> (17.946, -33.5433)
  line L410 (12.464, -37.0385) -> (15.3479, -32.0433)
  line L411 (12.464, -40.0385) -> (15.3479, -45.0337)
  line L412 (43.33, -33.5433) -> (46.214, -33.5433)
  line L413 (43.33, -33.5433) -> (40.446, -33.5433)
  line L414 (48.8121, -32.0433) -> (51.696, -37.0385)
  line L415 (46.214, -33.5433) -> (49.0979, -38.5385)
  line L416 (40.446, -33.5433) -> (37.5621, -38.5385)
  line L417 (37.5621, -38.5385) -> (40.446, -43.5337)
  line L418 (40.446, -43.5337) -> (43.33, -43.5337)
  line L419 (46.214, -43.5337) -> (43.33, -43.5337)
  line L420 (49.0979, -38.5385) -> (46.214, -43.5337)
  line L421 (48.8121, -45.0337) -> (51.696, -40.0385)
  line L422 (-7.1521, -32.0433) -> (-10.036, -37.0385)
  line L423 (-7.1521, -45.0337) -> (-10.036, -40.0385)
  line L424 (-1.67, -33.5433) -> (-4.554, -33.5433)
  line L425 (-4.554, -33.5433) -> (-7.4379, -38.5385)
  line L426 (-7.4379, -38.5385) -> (-4.554, -43.5337)
  line L427 (-4.554, -43.5337) -> (-1.67, -43.5337)
  line L428 (3.8121, -45.0337) -> (6.696, -40.0385)
  line L429 (4.0979, -38.5385) -> (1.214, -43.5337)
  line L430 (-1.67, -33.5433) -> (1.214, -33.5433)
  line L431 (1.214, -33.5433) -> (4.0979, -38.5385)
  line L432 (1.214, -43.5337) -> (-1.67, -43.5337)
  line L433 (3.8121, -32.0433) -> (6.696, -37.0385)
  line L434 (-29.9379, -38.5385) -> (-27.054, -43.5337)
  line L435 (-27.054, -43.5337) -> (-21.286, -43.5337)
  line L436 (-21.286, -43.5337) -> (-18.4021, -38.5385)
  line L437 (-10.036, -37.0385) -> (-15.804, -37.0385)
  line L438 (-15.804, -37.0385) -> (-18.6879, -32.0433)
  line L439 (-15.804, -40.0385) -> (-18.6879, -45.0337)
  line L440 (-10.036, -40.0385) -> (-15.804, -40.0385)
  line L441 (46.214, -20.5529) -> (43.33, -20.5529)
  line L442 (48.8121, -19.0529) -> (51.696, -24.0481)
  line L443 (49.0979, -25.5481) -> (46.214, -20.5529)
  line L444 (37.5621, -25.5481) -> (40.446, -20.5529)
  line L445 (40.446, -20.5529) -> (43.33, -20.5529)
  line L446 (-1.67, -30.5433) -> (1.214, -30.5433)
  line L447 (-1.67, -30.5433) -> (-4.554, -30.5433)
  line L448 (3.8121, -32.0433) -> (6.696, -27.0481)
  line L449 (1.214, -30.5433) -> (4.0979, -25.5481)
  line L450 (-7.1521, -32.0433) -> (-10.036, -27.0481)
  line L451 (-4.554, -30.5433) -> (-7.4379, -25.5481)
  line L452 (4.0979, -25.5481) -> (1.214, -20.5529)
  line L453 (1.214, -20.5529) -> (-1.67, -20.5529)
  line L454 (-4.554, -20.5529) -> (-1.67, -20.5529)
  line L455 (-10.036, -27.0481) -> (-15.804, -27.0481)
  line L456 (-10.036, -24.0481) -> (-15.804, -24.0481)
  line L457 (-7.4379, -25.5481) -> (-4.554, -20.5529)
  line L458 (-7.1521, -19.0529) -> (-10.036, -24.0481)
  line L459 (3.8121, -19.0529) -> (6.696, -24.0481)
  line L460 (60.0621, -38.5385) -> (62.946, -33.5433)
  line L461 (57.464, -37.0385) -> (60.3479, -32.0433)
  line L462 (62.946, -43.5337) -> (60.0621, -38.5385)
  line L463 (57.464, -40.0385) -> (60.3479, -45.0337)
  line L464 (51.696, -40.0385) -> (57.464, -40.0385)
  line L465 (51.696, -37.0385) -> (57.464, -37.0385)
  line L466 (51.696, -27.0481) -> (57.464, -27.0481)
  line L467 (51.696, -24.0481) -> (57.464, -24.0481)
  line L468 (57.464, -27.0481) -> (60.3479, -32.0433)
  line L469 (60.0621, -25.5481) -> (62.946, -30.5433)
  line L470 (62.946, -20.5529) -> (60.0621, -25.5481)
  line L471 (57.464, -24.0481) -> (60.3479, -19.0529)
  line L472 (23.714, -30.5433) -> (20.83, -30.5433)
  line L473 (29.196, -27.0481) -> (26.3121, -32.0433)
  line L474 (26.5979, -25.5481) -> (23.714, -30.5433)
  line L475 (34.964, -27.0481) -> (29.196, -27.0481)
  line L476 (20.83, -20.5529) -> (23.714, -20.5529)
  line L477 (23.714, -20.5529) -> (26.5979, -25.5481)
  line L478 (34.964, -24.0481) -> (29.196, -24.0481)
  line L479 (29.196, -24.0481) -> (26.3121, -19.0529)
  line L480 (37.8479, -19.0529) -> (34.964, -24.0481)
  line L481 (37.8479, -32.0433) -> (34.964, -27.0481)
  line L482 (6.696, -40.0385) -> (12.464, -40.0385)
  line L483 (6.696, -37.0385) -> (12.464, -37.0385)
  line L484 (6.696, -27.0481) -> (12.464, -27.0481)
  line L485 (6.696, -24.0481) -> (12.464, -24.0481)
  line L486 (12.464, -24.0481) -> (15.3479, -19.0529)
  line L487 (12.464, -27.0481) -> (15.3479, -32.0433)
  line L488 (17.946, -20.5529) -> (15.0621, -25.5481)
  line L489 (20.83, -20.5529) -> (17.946, -20.5529)
  line L490 (15.0621, -25.5481) -> (17.946, -30.5433)
  line L491 (17.946, -30.5433) -> (20.83, -30.5433)
  line L492 (-29.9379, -25.5481) -> (-27.054, -20.5529)
  line L493 (-33.4021, -25.5481) -> (-29.6521, -19.0529)
  line L494 (-27.054, -20.5529) -> (-21.286, -20.5529)
  line L495 (-21.286, -20.5529) -> (-18.4021, -25.5481)
  line L496 (-15.804, -24.0481) -> (-18.6879, -19.0529)
  line L497 (48.8121, -32.0433) -> (51.696, -27.0481)
  line L498 (43.33, -30.5433) -> (40.446, -30.5433)
  line L499 (46.214, -30.5433) -> (49.0979, -25.5481)
  line L500 (40.446, -30.5433) -> (37.5621, -25.5481)
  line L501 (43.33, -30.5433) -> (46.214, -30.5433)
  line L502 (-21.286, 99.3605) -> (-27.054, 99.3605)
  line L503 (-27.054, 99.3605) -> (-29.9379, 104.3557)
  line L504 (-29.9379, 104.3557) -> (-27.054, 109.3509)
  line L505 (-27.054, 109.3509) -> (-21.286, 109.3509)
  line L506 (-21.286, 109.3509) -> (-18.4021, 104.3557)
  line L507 (-18.4021, 104.3557) -> (-21.286, 99.3605)
  line L508 (-7.1521, 97.8605) -> (-10.036, 102.8557)
  line L509 (-10.036, 102.8557) -> (-15.804, 102.8557)
  line L510 (-15.804, 102.8557) -> (-18.6879, 97.8605)
  line L511 (-7.1521, 110.8509) -> (-10.036, 105.8557)
  line L512 (-10.036, 105.8557) -> (-15.804, 105.8557)
  line L513 (-15.804, 105.8557) -> (-18.6879, 110.8509)
  line L514 (-1.67, 99.3605) -> (-4.554, 99.3605)
  line L515 (-4.554, 99.3605) -> (-7.4379, 104.3557)
  line L516 (-7.4379, 104.3557) -> (-4.554, 109.3509)
  line L517 (-4.554, 109.3509) -> (-1.67, 109.3509)
  line L518 (3.8121, 110.8509) -> (6.696, 105.8557)
  line L519 (4.0979, 104.3557) -> (1.214, 109.3509)
  line L520 (-1.67, 99.3605) -> (1.214, 99.3605)
  line L521 (1.214, 99.3605) -> (4.0979, 104.3557)
  line L522 (3.8121, 97.8605) -> (6.696, 102.8557)
  line L523 (6.696, 105.8557) -> (12.464, 105.8557)
  line L524 (6.696, 102.8557) -> (12.464, 102.8557)
  line L525 (12.464, 105.8557) -> (15.3479, 110.8509)
  line L526 (1.214, 109.3509) -> (-1.67, 109.3509)
  line L527 (17.946, 109.3509) -> (15.0621, 104.3557)
  line L528 (12.464, 102.8557) -> (15.3479, 97.8605)
  line L529 (15.0621, 104.3557) -> (17.946, 99.3605)
  line L530 (17.946, 99.3605) -> (20.83, 99.3605)
  line L531 (20.83, 109.3509) -> (17.946, 109.3509)
  line L532 (23.714, 99.3605) -> (20.83, 99.3605)
  line L533 (60.0621, 104.3557) -> (62.946, 99.3605)
  line L534 (57.464, 102.8557) -> (60.3479, 97.8605)
  line L535 (62.946, 109.3509) -> (60.0621, 104.3557)
  line L536 (57.464, 105.8557) -> (60.3479, 110.8509)
  line L537 (51.696, 105.8557) -> (57.464, 105.8557)
  line L538 (51.696, 102.8557) -> (57.464, 102.8557)
  line L539 (37.8479, 110.8509) -> (34.964, 105.8557)
  line L540 (34.964, 105.8557) -> (29.196, 105.8557)
  line L541 (34.964, 102.8557) -> (29.196, 102.8557)
  line L542 (37.8479, 97.8605) -> (34.964, 102.8557)
  line L543 (40.446, 99.3605) -> (37.5621, 104.3557)
  line L544 (37.5621, 104.3557) -> (40.446, 109.3509)
  line L545 (43.33, 99.3605) -> (40.446, 99.3605)
  line L546 (20.83, 109.3509) -> (23.714, 109.3509)
  line L547 (29.196, 105.8557) -> (26.3121, 110.8509)
  line L548 (23.714, 109.3509) -> (26.5979, 104.3557)
  line L549 (29.196, 102.8557) -> (26.3121, 97.8605)
  line L550 (26.5979, 104.3557) -> (23.714, 99.3605)
  line L551 (48.8121, 97.8605) -> (51.696, 102.8557)
  line L552 (48.8121, 110.8509) -> (51.696, 105.8557)
  line L553 (46.214, 99.3605) -> (49.0979, 104.3557)
  line L554 (49.0979, 104.3557) -> (46.214, 109.3509)
  line L555 (46.214, 109.3509) -> (43.33, 109.3509)
  line L556 (40.446, 109.3509) -> (43.33, 109.3509)
  line L557 (43.33, 99.3605) -> (46.214, 99.3605)
  line L558 (-18.4021, 91.3653) -> (-21.286, 96.3605)
  line L559 (-21.286, 86.3701) -> (-18.4021, 91.3653)
  line L560 (-27.054, 86.3701) -> (-21.286, 86.3701)
  line L561 (-21.286, 96.3605) -> (-27.054, 96.3605)
  line L562 (-15.804, 89.8653) -> (-18.6879, 84.8701)
  line L563 (-10.036, 89.8653) -> (-15.804, 89.8653)
  line L564 (-10.036, 92.8653) -> (-15.804, 92.8653)
  line L565 (-7.1521, 84.8701) -> (-10.036, 89.8653)
  line L566 (-7.4379, 91.3653) -> (-4.554, 86.3701)
  line L567 (-7.1521, 97.8605) -> (-10.036, 92.8653)
  line L568 (-4.554, 96.3605) -> (-7.4379, 91.3653)
  line L569 (-15.804, 92.8653) -> (-18.6879, 97.8605)
  line L570 (-1.67, 96.3605) -> (-4.554, 96.3605)
  line L571 (-4.554, 86.3701) -> (-1.67, 86.3701)
  line L572 (1.214, 86.3701) -> (-1.67, 86.3701)
  line L573 (-1.67, 96.3605) -> (1.214, 96.3605)
  line L574 (4.0979, 91.3653) -> (1.214, 86.3701)
  line L575 (3.8121, 84.8701) -> (6.696, 89.8653)
  line L576 (1.214, 96.3605) -> (4.0979, 91.3653)
  line L577 (3.8121, 97.8605) -> (6.696, 92.8653)
  line L578 (17.946, 96.3605) -> (20.83, 96.3605)
  line L579 (12.464, 92.8653) -> (15.3479, 97.8605)
  line L580 (6.696, 92.8653) -> (12.464, 92.8653)
  line L581 (15.0621, 91.3653) -> (17.946, 96.3605)
  line L582 (6.696, 89.8653) -> (12.464, 89.8653)
  line L583 (17.946, 86.3701) -> (15.0621, 91.3653)
  line L584 (12.464, 89.8653) -> (15.3479, 84.8701)
  line L585 (20.83, 86.3701) -> (17.946, 86.3701)
  line L586 (51.696, 92.8653) -> (57.464, 92.8653)
  line L587 (51.696, 89.8653) -> (57.464, 89.8653)
  line L588 (20.83, 86.3701) -> (23.714, 86.3701)
  line L589 (23.714, 96.3605) -> (20.83, 96.3605)
  line L590 (23.714, 86.3701) -> (26.5979, 91.3653)
  line L591 (26.5979, 91.3653) -> (23.714, 96.3605)
  line L592 (29.196, 92.8653) -> (26.3121, 97.8605)
  line L593 (29.196, 89.8653) -> (26.3121, 84.8701)
  line L594 (34.964, 92.8653) -> (29.196, 92.8653)
  line L595 (34.964, 89.8653) -> (29.196, 89.8653)
  line L596 (37.8479, 97.8605) -> (34.964, 92.8653)
  line L597 (37.8479, 84.8701) -> (34.964, 89.8653)
  line L598 (48.8121, 84.8701) -> (51.696, 89.8653)
  line L599 (48.8121, 97.8605) -> (51.696, 92.8653)
  line L600 (46.214, 96.3605) -> (49.0979, 91.3653)
  line L601 (49.0979, 91.3653) -> (46.214, 86.3701)
  line L602 (43.33, 96.3605) -> (46.214, 96.3605)
  line L603 (46.214, 86.3701) -> (43.33, 86.3701)
  line L604 (43.33, 96.3605) -> (40.446, 96.3605)
  line L605 (40.446, 96.3605) -> (37.5621, 91.3653)
  line L606 (40.446, 86.3701) -> (43.33, 86.3701)
  line L607 (37.5621, 91.3653) -> (40.446, 86.3701)
  line L608 (57.464, 89.8653) -> (60.3479, 84.8701)
  line L609 (57.464, 92.8653) -> (60.3479, 97.8605)
  line L610 (60.0621, 91.3653) -> (62.946, 96.3605)
  line L611 (62.946, 86.3701) -> (60.0621, 91.3653)
  line L612 (-27.054, 96.3605) -> (-29.9379, 91.3653)
  line L613 (-29.9379, 91.3653) -> (-27.054, 86.3701)
  line L614 (-32.969, 103.6057) -> (-29.6521, 97.8605)
  line L615 (-29.6521, 97.8605) -> (-33.4021, 91.3653)
  line L616 (-33.4021, 91.3653) -> (-29.6521, 84.8701)
  line L617 (-15.804, 76.875) -> (-18.6879, 71.8798)
  line L618 (-18.4021, 78.375) -> (-21.286, 73.3798)
  line L619 (-21.286, 73.3798) -> (-27.054, 73.3798)
  line L620 (-18.4021, 65.3846) -> (-21.286, 70.3798)
  line L621 (-27.054, 73.3798) -> (-29.9379, 78.375)
  line L622 (-29.6521, 71.8798) -> (-33.4021, 78.375)
  line L623 (-32.969, 66.1346) -> (-29.6521, 71.8798)
  line L624 (-27.054, 70.3798) -> (-29.9379, 65.3846)
  line L625 (-21.286, 70.3798) -> (-27.054, 70.3798)
  line L626 (23.714, 60.3894) -> (26.5979, 65.3846)
  line L627 (26.5979, 65.3846) -> (23.714, 70.3798)
  line L628 (29.196, 63.8846) -> (26.3121, 58.8894)
  line L629 (29.196, 66.8846) -> (26.3121, 71.8798)
  line L630 (34.964, 66.8846) -> (29.196, 66.8846)
  line L631 (34.964, 63.8846) -> (29.196, 63.8846)
  line L632 (37.8479, 71.8798) -> (34.964, 66.8846)
  line L633 (37.8479, 58.8894) -> (34.964, 63.8846)
  line L634 (23.714, 70.3798) -> (20.83, 70.3798)
  line L635 (20.83, 60.3894) -> (23.714, 60.3894)
  line L636 (20.83, 60.3894) -> (17.946, 60.3894)
  line L637 (17.946, 70.3798) -> (20.83, 70.3798)
  line L638 (17.946, 60.3894) -> (15.0621, 65.3846)
  line L639 (15.0621, 65.3846) -> (17.946, 70.3798)
  line L640 (12.464, 66.8846) -> (15.3479, 71.8798)
  line L641 (12.464, 63.8846) -> (15.3479, 58.8894)
  line L642 (43.33, 70.3798) -> (46.214, 70.3798)
  line L643 (43.33, 70.3798) -> (40.446, 70.3798)
  line L644 (48.8121, 71.8798) -> (51.696, 66.8846)
  line L645 (46.214, 70.3798) -> (49.0979, 65.3846)
  line L646 (40.446, 70.3798) -> (37.5621, 65.3846)
  line L647 (37.5621, 65.3846) -> (40.446, 60.3894)
  line L648 (40.446, 60.3894) -> (43.33, 60.3894)
  line L649 (46.214, 60.3894) -> (43.33, 60.3894)
  line L650 (49.0979, 65.3846) -> (46.214, 60.3894)
  line L651 (48.8121, 58.8894) -> (51.696, 63.8846)
  line L652 (-7.1521, 71.8798) -> (-10.036, 66.8846)
  line L653 (-7.1521, 58.8894) -> (-10.036, 63.8846)
  line L654 (-1.67, 70.3798) -> (-4.554, 70.3798)
  line L655 (-4.554, 70.3798) -> (-7.4379, 65.3846)
  line L656 (-7.4379, 65.3846) -> (-4.554, 60.3894)
  line L657 (-4.554, 60.3894) -> (-1.67, 60.3894)
  line L658 (3.8121, 58.8894) -> (6.696, 63.8846)
  line L659 (4.0979, 65.3846) -> (1.214, 60.3894)
  line L660 (-1.67, 70.3798) -> (1.214, 70.3798)
  line L661 (1.214, 70.3798) -> (4.0979, 65.3846)
  line L662 (1.214, 60.3894) -> (-1.67, 60.3894)
  line L663 (3.8121, 71.8798) -> (6.696, 66.8846)
  line L664 (-29.9379, 65.3846) -> (-27.054, 60.3894)
  line L665 (-27.054, 60.3894) -> (-21.286, 60.3894)
  line L666 (-21.286, 60.3894) -> (-18.4021, 65.3846)
  line L667 (-10.036, 66.8846) -> (-15.804, 66.8846)
  line L668 (-15.804, 66.8846) -> (-18.6879, 71.8798)
  line L669 (-15.804, 63.8846) -> (-18.6879, 58.8894)
  line L670 (-10.036, 63.8846) -> (-15.804, 63.8846)
  line L671 (46.214, 83.3701) -> (43.33, 83.3701)
  line L672 (48.8121, 84.8701) -> (51.696, 79.875)
  line L673 (49.0979, 78.375) -> (46.214, 83.3701)
  line L674 (37.5621, 78.375) -> (40.446, 83.3701)
  line L675 (40.446, 83.3701) -> (43.33, 83.3701)
  line L676 (-1.67, 73.3798) -> (1.214, 73.3798)
  line L677 (-1.67, 73.3798) -> (-4.554, 73.3798)
  line L678 (3.8121, 71.8798) -> (6.696, 76.875)
  line L679 (1.214, 73.3798) -> (4.0979, 78.375)